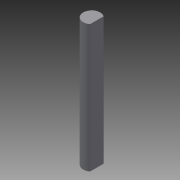
# Autodesk Inventor part: DMJ_arm
Saved by Autodesk Inventor 2015 SP1 (Build 190203100, 203)
## iProperties
Created: 2016-02-03
Part Number: DMJ_arm
Material: Generic
Document SubType Name: Modeling
Designer: guillemd
Density: 0.916182 g/cm^3
Appearance: Default
Mass: 11339.8 g
Surface Area: 3862.01 cm^2
Volume: 12377.2 cm^3
Author: guillemd
Autodesk Inventor part; units mm, degrees
ref_plane "YZ Plane" through (0, 0, 0) normal (1, 0, 0) x (0, 1, 0)
ref_plane "XZ Plane" through (0, 0, 0) normal (0, 1, 0) x (-1, 0, 0)
ref_plane "XY Plane" through (0, 0, 0) normal (0, 0, 1) x (1, 0, 0)
sketch "Sketch1" plane through (0, 0, 0) normal (0, 1, 0) x (-1, 0, 0)
  arc A0 (0, -40.64) -> (0, 40.64) centre (30.48, 0) ccw
  line L0 (0, -71.12) -> (0, 71.12) projected
  line L1 (97.536, 0) -> (-16.256, 0) projected
  line L2 (0, 40.64) -> (0, -40.64)
  point P0 (0, 0)
  point P1 (81.28, 0)
  dimension "d0" = 50.8
  dimension "d4" = 30.48
  constraints: 3 point on circle, 3 point on line, 2 end point, 1 centre point, 1 collinear
  measures "d0" radius of A0
  measures "d4" distance from line of L0 A0.centre
extrude "Extrusion1" add sketch "Sketch1" along normal blind 762
body "Solid1"
